Autodesk Inventor part; units mm, degrees
(part 2 of 2)
sketch "Sketch4" plane through (0, 0, -2.75) normal (0, 0, -1) x (-1, 0, 0)
  arc A0 (0.3991, 3.7387) -> (0.581, 3.8546) centre (0.3991, 3.9394) ccw
  line L0 (0.581, 3.8546) -> (0.7391, 4.1936)
  arc A1 (1.0847, 4.3585) -> (0.7391, 4.1936) centre (1.012, 4.0663) ccw
  arc A2 (1.2398, 4.317) -> (1.0847, 4.3585) centre (0, 0) ccw
  arc A3 (1.4567, 4.0013) -> (1.2398, 4.317) centre (1.1567, 4.0275) ccw
  line L1 (1.4567, 4.0013) -> (1.4241, 3.6287)
  arc A4 (1.4241, 3.6287) -> (1.5237, 3.4373) centre (1.6241, 3.6112) ccw
  line L2 (1.5237, 3.4373) -> (2.2149, 3.0382)
  arc A5 (2.2149, 3.0382) -> (2.4305, 3.0476) centre (2.3153, 3.2121) ccw
  line L3 (2.4305, 3.0476) -> (2.7369, 3.2622)
  arc A6 (3.1187, 3.2322) -> (2.7369, 3.2622) centre (2.9096, 3.0155) ccw
  arc A7 (3.2322, 3.1187) -> (3.1187, 3.2322) centre (0, 0) ccw
  arc A8 (3.2622, 2.7369) -> (3.2322, 3.1187) centre (3.0155, 2.9096) ccw
  line L4 (3.2622, 2.7369) -> (3.0476, 2.4305)
  arc A9 (3.0476, 2.4305) -> (3.0382, 2.2149) centre (3.2121, 2.3153) ccw
  line L5 (3.0382, 2.2149) -> (3.4373, 1.5237)
  arc A10 (3.4373, 1.5237) -> (3.6287, 1.4241) centre (3.6112, 1.6241) ccw
  line L6 (3.6287, 1.4241) -> (4.0013, 1.4567)
  arc A11 (4.317, 1.2398) -> (4.0013, 1.4567) centre (4.0275, 1.1567) ccw
  arc A12 (4.3585, 1.0847) -> (4.317, 1.2398) centre (0, 0) ccw
  arc A13 (4.1936, 0.7391) -> (4.3585, 1.0847) centre (4.0663, 1.012) ccw
  line L7 (4.1936, 0.7391) -> (3.8546, 0.581)
  arc A14 (3.8546, 0.581) -> (3.7387, 0.3991) centre (3.9394, 0.3991) ccw
  line L8 (3.7387, 0.3991) -> (3.7387, -0.3991)
  arc A15 (3.7387, -0.3991) -> (3.8546, -0.581) centre (3.9394, -0.3991) ccw
  line L9 (3.8546, -0.581) -> (4.1936, -0.7391)
  arc A16 (4.3585, -1.0847) -> (4.1936, -0.7391) centre (4.0663, -1.012) ccw
  arc A17 (4.317, -1.2398) -> (4.3585, -1.0847) centre (0, 0) ccw
  arc A18 (4.0013, -1.4567) -> (4.317, -1.2398) centre (4.0275, -1.1567) ccw
  line L10 (4.0013, -1.4567) -> (3.6287, -1.4241)
  arc A19 (3.6287, -1.4241) -> (3.4373, -1.5237) centre (3.6112, -1.6241) ccw
  line L11 (3.4373, -1.5237) -> (3.0382, -2.2149)
  arc A20 (3.0382, -2.2149) -> (3.0476, -2.4305) centre (3.2121, -2.3153) ccw
  line L12 (3.0476, -2.4305) -> (3.2622, -2.7369)
  arc A21 (3.2322, -3.1187) -> (3.2622, -2.7369) centre (3.0155, -2.9096) ccw
  arc A22 (3.1187, -3.2322) -> (3.2322, -3.1187) centre (0, 0) ccw
  arc A23 (2.7369, -3.2622) -> (3.1187, -3.2322) centre (2.9096, -3.0155) ccw
  line L13 (2.7369, -3.2622) -> (2.4305, -3.0476)
  arc A24 (2.4305, -3.0476) -> (2.2149, -3.0382) centre (2.3153, -3.2121) ccw
  line L14 (2.2149, -3.0382) -> (1.5237, -3.4373)
  arc A25 (1.5237, -3.4373) -> (1.4241, -3.6287) centre (1.6241, -3.6112) ccw
  line L15 (1.4241, -3.6287) -> (1.4567, -4.0013)
  arc A26 (1.2398, -4.317) -> (1.4567, -4.0013) centre (1.1567, -4.0275) ccw
  arc A27 (1.0847, -4.3585) -> (1.2398, -4.317) centre (0, 0) ccw
  arc A28 (0.7391, -4.1936) -> (1.0847, -4.3585) centre (1.012, -4.0663) ccw
  line L16 (0.7391, -4.1936) -> (0.581, -3.8546)
  arc A29 (0.581, -3.8546) -> (0.3991, -3.7387) centre (0.3991, -3.9394) ccw
  line L17 (0.3991, -3.7387) -> (-0.3991, -3.7387)
  arc A30 (-0.3991, -3.7387) -> (-0.581, -3.8546) centre (-0.3991, -3.9394) ccw
  line L18 (-0.581, -3.8546) -> (-0.7391, -4.1936)
  arc A31 (-1.0847, -4.3585) -> (-0.7391, -4.1936) centre (-1.012, -4.0663) ccw
  arc A32 (-1.2398, -4.317) -> (-1.0847, -4.3585) centre (0, 0) ccw
  arc A33 (-1.4567, -4.0013) -> (-1.2398, -4.317) centre (-1.1567, -4.0275) ccw
  line L19 (-1.4567, -4.0013) -> (-1.4241, -3.6287)
  arc A34 (-1.4241, -3.6287) -> (-1.5237, -3.4373) centre (-1.6241, -3.6112) ccw
  line L20 (-1.5237, -3.4373) -> (-2.2149, -3.0382)
  arc A35 (-2.2149, -3.0382) -> (-2.4305, -3.0476) centre (-2.3153, -3.2121) ccw
  line L21 (-2.4305, -3.0476) -> (-2.7369, -3.2622)
  arc A36 (-3.1187, -3.2322) -> (-2.7369, -3.2622) centre (-2.9096, -3.0155) ccw
  arc A37 (-3.2322, -3.1187) -> (-3.1187, -3.2322) centre (0, 0) ccw
  arc A38 (-3.2622, -2.7369) -> (-3.2322, -3.1187) centre (-3.0155, -2.9096) ccw
  line L22 (-3.2622, -2.7369) -> (-3.0476, -2.4305)
  arc A39 (-3.0476, -2.4305) -> (-3.0382, -2.2149) centre (-3.2121, -2.3153) ccw
  line L23 (-3.0382, -2.2149) -> (-3.4373, -1.5237)
  arc A40 (-3.4373, -1.5237) -> (-3.6287, -1.4241) centre (-3.6112, -1.6241) ccw
  line L24 (-3.6287, -1.4241) -> (-4.0013, -1.4567)
  arc A41 (-4.317, -1.2398) -> (-4.0013, -1.4567) centre (-4.0275, -1.1567) ccw
  arc A42 (-4.3585, -1.0847) -> (-4.317, -1.2398) centre (0, 0) ccw
  arc A43 (-4.1936, -0.7391) -> (-4.3585, -1.0847) centre (-4.0663, -1.012) ccw
  line L25 (-4.1936, -0.7391) -> (-3.8546, -0.581)
  arc A44 (-3.8546, -0.581) -> (-3.7387, -0.3991) centre (-3.9394, -0.3991) ccw
  line L26 (-3.7387, -0.3991) -> (-3.7387, 0.3991)
  arc A45 (-3.7387, 0.3991) -> (-3.8546, 0.581) centre (-3.9394, 0.3991) ccw
  line L27 (-3.8546, 0.581) -> (-4.1936, 0.7391)
  arc A46 (-4.3585, 1.0847) -> (-4.1936, 0.7391) centre (-4.0663, 1.012) ccw
  arc A47 (-4.317, 1.2398) -> (-4.3585, 1.0847) centre (0, 0) ccw
  arc A48 (-4.0013, 1.4567) -> (-4.317, 1.2398) centre (-4.0275, 1.1567) ccw
  line L28 (-4.0013, 1.4567) -> (-3.6287, 1.4241)
  arc A49 (-3.6287, 1.4241) -> (-3.4373, 1.5237) centre (-3.6112, 1.6241) ccw
  line L29 (-3.4373, 1.5237) -> (-3.0382, 2.2149)
  arc A50 (-3.0382, 2.2149) -> (-3.0476, 2.4305) centre (-3.2121, 2.3153) ccw
  line L30 (-3.0476, 2.4305) -> (-3.2622, 2.7369)
  arc A51 (-3.2322, 3.1187) -> (-3.2622, 2.7369) centre (-3.0155, 2.9096) ccw
  arc A52 (-3.1187, 3.2322) -> (-3.2322, 3.1187) centre (0, 0) ccw
  arc A53 (-2.7369, 3.2622) -> (-3.1187, 3.2322) centre (-2.9096, 3.0155) ccw
  line L31 (-2.7369, 3.2622) -> (-2.4305, 3.0476)
  arc A54 (-2.4305, 3.0476) -> (-2.2149, 3.0382) centre (-2.3153, 3.2121) ccw
  line L32 (-2.2149, 3.0382) -> (-1.5237, 3.4373)
  arc A55 (-1.5237, 3.4373) -> (-1.4241, 3.6287) centre (-1.6241, 3.6112) ccw
  line L33 (-1.4241, 3.6287) -> (-1.4567, 4.0013)
  arc A56 (-1.2398, 4.317) -> (-1.4567, 4.0013) centre (-1.1567, 4.0275) ccw
  arc A57 (-1.0847, 4.3585) -> (-1.2398, 4.317) centre (0, 0) ccw
  arc A58 (-0.7391, 4.1936) -> (-1.0847, 4.3585) centre (-1.012, 4.0663) ccw
  line L34 (-0.7391, 4.1936) -> (-0.581, 3.8546)
  arc A59 (-0.581, 3.8546) -> (-0.3991, 3.7387) centre (-0.3991, 3.9394) ccw
  line L35 (-0.3991, 3.7387) -> (0.3991, 3.7387)
  circle A60 centre (0, 0) radius 6.84
  arc A61 (1.5737, -3.5239) -> (1.5237, -3.6199) centre (1.6241, -3.6112) ccw
  line L36 (1.5737, -3.5239) -> (2.2649, -3.1248)
  arc A62 (2.3731, -3.1296) -> (2.2649, -3.1248) centre (2.3153, -3.2121) ccw
  line L37 (2.3731, -3.1296) -> (2.6795, -3.3441)
  arc A63 (2.6795, -3.3441) -> (3.1881, -3.3042) centre (2.9096, -3.0155) ccw
  arc A64 (3.1881, -3.3042) -> (3.3042, -3.1881) centre (0, 0) ccw
  arc A65 (3.3042, -3.1881) -> (3.3441, -2.6795) centre (3.0155, -2.9096) ccw
  line L38 (3.3441, -2.6795) -> (3.1296, -2.3731)
  arc A66 (3.1248, -2.2649) -> (3.1296, -2.3731) centre (3.2121, -2.3153) ccw
  line L39 (3.1248, -2.2649) -> (3.5239, -1.5737)
  arc A67 (3.6199, -1.5237) -> (3.5239, -1.5737) centre (3.6112, -1.6241) ccw
  line L40 (3.6199, -1.5237) -> (3.9926, -1.5563)
  arc A68 (3.9926, -1.5563) -> (4.4131, -1.2674) centre (4.0275, -1.1567) ccw
  arc A69 (4.4131, -1.2674) -> (4.4556, -1.1089) centre (0, 0) ccw
  arc A70 (4.4556, -1.1089) -> (4.2358, -0.6485) centre (4.0663, -1.012) ccw
  line L41 (4.2358, -0.6485) -> (3.8968, -0.4904)
  arc A71 (3.8387, -0.3991) -> (3.8968, -0.4904) centre (3.9394, -0.3991) ccw
  line L42 (3.8387, -0.3991) -> (3.8387, 0.3991)
  arc A72 (3.8968, 0.4904) -> (3.8387, 0.3991) centre (3.9394, 0.3991) ccw
  line L43 (3.8968, 0.4904) -> (4.2358, 0.6485)
  arc A73 (4.2358, 0.6485) -> (4.4556, 1.1089) centre (4.0663, 1.012) ccw
  arc A74 (4.4556, 1.1089) -> (4.4131, 1.2674) centre (0, 0) ccw
  arc A75 (4.4131, 1.2674) -> (3.9926, 1.5563) centre (4.0275, 1.1567) ccw
  line L44 (3.9926, 1.5563) -> (3.6199, 1.5237)
  arc A76 (3.5239, 1.5737) -> (3.6199, 1.5237) centre (3.6112, 1.6241) ccw
  line L45 (3.5239, 1.5737) -> (3.1248, 2.2649)
  arc A77 (3.1296, 2.3731) -> (3.1248, 2.2649) centre (3.2121, 2.3153) ccw
  line L46 (3.1296, 2.3731) -> (3.3441, 2.6795)
  arc A78 (3.3441, 2.6795) -> (3.3042, 3.1881) centre (3.0155, 2.9096) ccw
  arc A79 (3.3042, 3.1881) -> (3.1881, 3.3042) centre (0, 0) ccw
  arc A80 (3.1881, 3.3042) -> (2.6795, 3.3441) centre (2.9096, 3.0155) ccw
  line L47 (2.6795, 3.3441) -> (2.3731, 3.1296)
  arc A81 (2.2649, 3.1248) -> (2.3731, 3.1296) centre (2.3153, 3.2121) ccw
  line L48 (2.2649, 3.1248) -> (1.5737, 3.5239)
  arc A82 (1.5237, 3.6199) -> (1.5737, 3.5239) centre (1.6241, 3.6112) ccw
  line L49 (1.5237, 3.6199) -> (1.5563, 3.9926)
  arc A83 (1.5563, 3.9926) -> (1.2674, 4.4131) centre (1.1567, 4.0275) ccw
  arc A84 (1.2674, 4.4131) -> (1.1089, 4.4556) centre (0, 0) ccw
  arc A85 (1.1089, 4.4556) -> (0.6485, 4.2358) centre (1.012, 4.0663) ccw
  line L50 (0.6485, 4.2358) -> (0.4904, 3.8968)
  arc A86 (0.3991, 3.8387) -> (0.4904, 3.8968) centre (0.3991, 3.9394) ccw
  line L51 (0.3991, 3.8387) -> (-0.3991, 3.8387)
  arc A87 (-0.4904, 3.8968) -> (-0.3991, 3.8387) centre (-0.3991, 3.9394) ccw
  line L52 (-0.4904, 3.8968) -> (-0.6485, 4.2358)
  arc A88 (-0.6485, 4.2358) -> (-1.1089, 4.4556) centre (-1.012, 4.0663) ccw
  arc A89 (-1.1089, 4.4556) -> (-1.2674, 4.4131) centre (0, 0) ccw
  arc A90 (-1.2674, 4.4131) -> (-1.5563, 3.9926) centre (-1.1567, 4.0275) ccw
  line L53 (-1.5563, 3.9926) -> (-1.5237, 3.6199)
  arc A91 (-1.5737, 3.5239) -> (-1.5237, 3.6199) centre (-1.6241, 3.6112) ccw
  line L54 (-1.5737, 3.5239) -> (-2.2649, 3.1248)
  arc A92 (-2.3731, 3.1296) -> (-2.2649, 3.1248) centre (-2.3153, 3.2121) ccw
  line L55 (-2.3731, 3.1296) -> (-2.6795, 3.3441)
  arc A93 (-2.6795, 3.3441) -> (-3.1881, 3.3042) centre (-2.9096, 3.0155) ccw
  arc A94 (-3.1881, 3.3042) -> (-3.3042, 3.1881) centre (0, 0) ccw
  arc A95 (-3.3042, 3.1881) -> (-3.3441, 2.6795) centre (-3.0155, 2.9096) ccw
  line L56 (-3.3441, 2.6795) -> (-3.1296, 2.3731)
  arc A96 (-3.1248, 2.2649) -> (-3.1296, 2.3731) centre (-3.2121, 2.3153) ccw
  line L57 (-3.1248, 2.2649) -> (-3.5239, 1.5737)
  arc A97 (-3.6199, 1.5237) -> (-3.5239, 1.5737) centre (-3.6112, 1.6241) ccw
  line L58 (-3.6199, 1.5237) -> (-3.9926, 1.5563)
  arc A98 (-3.9926, 1.5563) -> (-4.4131, 1.2674) centre (-4.0275, 1.1567) ccw
  arc A99 (-4.4131, 1.2674) -> (-4.4556, 1.1089) centre (0, 0) ccw
  arc A100 (-4.4556, 1.1089) -> (-4.2358, 0.6485) centre (-4.0663, 1.012) ccw
  line L59 (-4.2358, 0.6485) -> (-3.8968, 0.4904)
  arc A101 (-3.8387, 0.3991) -> (-3.8968, 0.4904) centre (-3.9394, 0.3991) ccw
  line L60 (-3.8387, 0.3991) -> (-3.8387, -0.3991)
  arc A102 (-3.8968, -0.4904) -> (-3.8387, -0.3991) centre (-3.9394, -0.3991) ccw
  line L61 (-3.8968, -0.4904) -> (-4.2358, -0.6485)
  arc A103 (-4.2358, -0.6485) -> (-4.4556, -1.1089) centre (-4.0663, -1.012) ccw
  arc A104 (-4.4556, -1.1089) -> (-4.4131, -1.2674) centre (0, 0) ccw
  arc A105 (-4.4131, -1.2674) -> (-3.9926, -1.5563) centre (-4.0275, -1.1567) ccw
  line L62 (-3.9926, -1.5563) -> (-3.6199, -1.5237)
  arc A106 (-3.5239, -1.5737) -> (-3.6199, -1.5237) centre (-3.6112, -1.6241) ccw
  line L63 (-3.5239, -1.5737) -> (-3.1248, -2.2649)
  arc A107 (-3.1296, -2.3731) -> (-3.1248, -2.2649) centre (-3.2121, -2.3153) ccw
  line L64 (-3.1296, -2.3731) -> (-3.3441, -2.6795)
  arc A108 (-3.3441, -2.6795) -> (-3.3042, -3.1881) centre (-3.0155, -2.9096) ccw
  arc A109 (-3.3042, -3.1881) -> (-3.1881, -3.3042) centre (0, 0) ccw
  arc A110 (-3.1881, -3.3042) -> (-2.6795, -3.3441) centre (-2.9096, -3.0155) ccw
  line L65 (-2.6795, -3.3441) -> (-2.3731, -3.1296)
  arc A111 (-2.2649, -3.1248) -> (-2.3731, -3.1296) centre (-2.3153, -3.2121) ccw
  line L66 (-2.2649, -3.1248) -> (-1.5737, -3.5239)
  arc A112 (-1.5237, -3.6199) -> (-1.5737, -3.5239) centre (-1.6241, -3.6112) ccw
  line L67 (-1.5237, -3.6199) -> (-1.5563, -3.9926)
  arc A113 (-1.5563, -3.9926) -> (-1.2674, -4.4131) centre (-1.1567, -4.0275) ccw
  arc A114 (-1.2674, -4.4131) -> (-1.1089, -4.4556) centre (0, 0) ccw
  arc A115 (-1.1089, -4.4556) -> (-0.6485, -4.2358) centre (-1.012, -4.0663) ccw
  line L68 (-0.6485, -4.2358) -> (-0.4904, -3.8968)
  arc A116 (-0.3991, -3.8387) -> (-0.4904, -3.8968) centre (-0.3991, -3.9394) ccw
  line L69 (-0.3991, -3.8387) -> (0.3991, -3.8387)
  arc A117 (0.4904, -3.8968) -> (0.3991, -3.8387) centre (0.3991, -3.9394) ccw
  line L70 (0.4904, -3.8968) -> (0.6485, -4.2358)
  arc A118 (0.6485, -4.2358) -> (1.1089, -4.4556) centre (1.012, -4.0663) ccw
  arc A119 (1.1089, -4.4556) -> (1.2674, -4.4131) centre (0, 0) ccw
  arc A120 (1.2674, -4.4131) -> (1.5563, -3.9926) centre (1.1567, -4.0275) ccw
  line L71 (1.5563, -3.9926) -> (1.5237, -3.6199)
  circle A121 centre (0, 0) radius 4.4915 construction
  dimension "d34" = 13.68
  dimension "d35" = 0.1
  constraints: 240 point on circle, 144 end point, 121 centre point, 2 coincident, 98 other
  measures "d34" diameter of A60
  measures "d35" radial gap between concentric circles of A25 A61
extrude "Extrusion7" add sketch "Sketch4" along normal blind 1 and the other way blind 0.5 contours A60
chamfer "Chamfer1" distance 2 distance2 1 1 edges at (6.84, 0, -3.75) measured on face at (6.34, 0, -3.75)
extrude "Extrusion4" cut sketch "Sketch4" against normal blind 3 contours A0 L0 A1 A2 A3 L1 A4 L2 A5 L3 A6 A7 A8 L4 A9 L5 A10 L6 A11 A12 A13 L7 A14 L8 A15 L9 A16 A17 A18 L10 A19 L11 A20 L12 A21 A22 A23 L13 A24 L14 A25 L15 A26 A27 A28 L16 A29 L17 A30 L18 A31 A32 A33 L19 A34 L20 A35 L21 A36 A37 A38 L22 A39 L23 A40 L24 A41 A42 A43 L25 A44 L26 A45 L27 A46 A47 A48 L28 A49 L29 A50 L30 A51 A52 A53 L31 A54 L32 A55 L33 A56 A57 A58 L34 A59 L35 | A61 L71 A120 A119 A118 L70 A117 L69 A116 L68 A115 A114 A113 L67 A112 L66 A111 L65 A110 A109 A108 L64 A107 L63 A106 L62 A105 A104 A103 L61 A102 L60 A101 L59 A100 A99 A98 L58 A97 L57 A96 L56 A95 A94 A93 L55 A92 L54 A91 L53 A90 A89 A88 L52 A87 L51 A86 L50 A85 A84 A83 L49 A82 L48 A81 L47 A80 A79 A78 L46 A77 L45 A76 L44 A75 A74 A73 L43 A72 L42 A71 L41 A70 A69 A68 L40 A67 L39 A66 L38 A65 A64 A63 L37 A62 L36
extrude "Extrusion5" add sketch "Sketch4" along normal blind 7.3 and the other way blind 2.8 from surface at 0 separate body contours A0 L0 A1 A2 A3 L1 A4 L2 A5 L3 A6 A7 A8 L4 A9 L5 A10 L6 A11 A12 A13 L7 A14 L8 A15 L9 A16 A17 A18 L10 A19 L11 A20 L12 A21 A22 A23 L13 A24 L14 A25 L15 A26 A27 A28 L16 A29 L17 A30 L18 A31 A32 A33 L19 A34 L20 A35 L21 A36 A37 A38 L22 A39 L23 A40 L24 A41 A42 A43 L25 A44 L26 A45 L27 A46 A47 A48 L28 A49 L29 A50 L30 A51 A52 A53 L31 A54 L32 A55 L33 A56 A57 A58 L34 A59 L35
extrude "Extrusion6" cut sketch "Sketch2" along normal through all both and the other way through all contours A1 bodies 2 1
equation "\"d1\" = da_a"
equation "\"d2\" = da_hg"
equation "\"d3\" = 2 * da_fi"
equation "\"d4\" = da_bw"
equation "\"d5\" = da_bf"
equation "\"d7\" = da_bf"
equation "\"d9\" = da_rb"
equation "\"d10\" = da_rt"
equation "\"da_pb\" = 2.5"
equation "\"da_fi\" = 25deg"
equation "\"da_hg\" = 0.75"
equation "\"da_bw\" = 1.05"
equation "\"da_rb\" = 0.2"
equation "\"da_rt\" = 0.3"
equation "\"da_a\" = 0.3"
equation "\"da_bf\" = 5.5"
equation "\"da_wf\" = 0.8"
equation "\"da_hf\" = 0.8"
